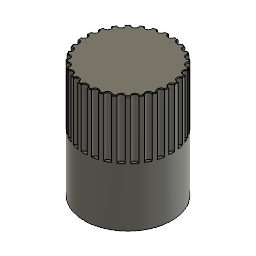
OpenMicroRotator (Autodesk Fusion 360 design; units mm, degrees)
Autodesk Fusion 360 part; units mm, degrees
sketch "Sketch1" plane through (0, 0, 0) normal (0, 1, 0) x (1, 0, 0)
  circle A0 centre (0, 0) radius 7.5
  dimension "d1" = 15
  constraint coincident A0.centre origin
  measures "d1" diameter of A0
extrude "Extrude1" add sketch "Sketch1" along normal blind 20
sketch "Sketch2" plane through (0, 0, 0) normal (0, -1, 0) x (1, 0, 0)
  circle A0 centre (0, 0) radius 7.5
  circle A1 centre (0, 0) radius 6.5
  dimension "d4" = 13
  constraint coincident A0.centre A1.centre
  measures "d4" diameter of A1
extrude "Extrude2" cut sketch "Sketch2" against normal blind 7 contours A1
sketch "Sketch3" plane through (0, 7, 0) normal (0, -1, 0) x (1, 0, 0)
  circle A0 centre (0, 0) radius 6.5
  circle A1 centre (0, 0) radius 3.025
  line L0 (-1.55, 2.5977) -> (-1.55, -2.5977)
  dimension "d7" = 6.05
  dimension "d8" = 1.55
  constraint coincident A0.centre A1.centre
  constraint coincident A1 L0.start
  constraint coincident A1 L0.end
  constraint vertical L0
  measures "d7" diameter of A1
  measures "d8" distance of A0.centre L0
extrude "Extrude3" cut sketch "Sketch3" against normal blind 10 contours A1 L0 picked at (0.0368, 0.8888)
sketch "Sketch4" plane through (0, 20, 0) normal (0, 1, 0) x (-1, 0, 0)
  circle A0 centre (0, 0) radius 7.5
  circle A1 centre (0, -7.5) radius 0.5
  circle A2 centre (1.6689, -7.312) radius 0.5
  circle A3 centre (3.2541, -6.7573) radius 0.5
  circle A4 centre (4.6762, -5.8637) radius 0.5
  circle A5 centre (5.8637, -4.6762) radius 0.5
  circle A6 centre (6.7573, -3.2541) radius 0.5
  circle A7 centre (7.312, -1.6689) radius 0.5
  circle A8 centre (7.5, 0) radius 0.5
  circle A9 centre (7.312, 1.6689) radius 0.5
  circle A10 centre (6.7573, 3.2541) radius 0.5
  circle A11 centre (5.8637, 4.6762) radius 0.5
  circle A12 centre (4.6762, 5.8637) radius 0.5
  circle A13 centre (3.2541, 6.7573) radius 0.5
  circle A14 centre (1.6689, 7.312) radius 0.5
  circle A15 centre (0, 7.5) radius 0.5
  circle A16 centre (-1.6689, 7.312) radius 0.5
  circle A17 centre (-3.2541, 6.7573) radius 0.5
  circle A18 centre (-4.6762, 5.8637) radius 0.5
  circle A19 centre (-5.8637, 4.6762) radius 0.5
  circle A20 centre (-6.7573, 3.2541) radius 0.5
  circle A21 centre (-7.312, 1.6689) radius 0.5
  circle A22 centre (-7.5, 0) radius 0.5
  circle A23 centre (-7.312, -1.6689) radius 0.5
  circle A24 centre (-6.7573, -3.2541) radius 0.5
  circle A25 centre (-5.8637, -4.6762) radius 0.5
  circle A26 centre (-4.6762, -5.8637) radius 0.5
  circle A27 centre (-3.2541, -6.7573) radius 0.5
  circle A28 centre (-1.6689, -7.312) radius 0.5
  dimension "d11" = 1
  dimension "d13" = 360
  constraint coincident A0 A1.centre
  measures "d11" diameter of A1
extrude "Extrude4" cut sketch "Sketch4" against normal blind 10 contours A0 A8 | A0 A9 | A0 A7 | A0 A10 | A0 A6 | A0 A11 | A0 A5 | A0 A12 | A0 A4 | A0 A13 | A0 A3 | A0 A14 | A0 A2 | A0 A15 | A0 A1 | A0 A16 | A0 A28 | A0 A17 | A0 A27 | A0 A18 | A0 A26 | A0 A19 | A0 A25 | A0 A20 | A0 A24 | A0 A21 | A0 A23 | A0 A22 picked at (7.3438, -0.1152) picked at (7.146, 1.6435) picked at (7.146, -1.6435) picked at (6.6117, 3.1705) picked at (6.6117, -3.1705) picked at (5.7404, 4.5622) picked at (5.7404, -4.5622) picked at (4.5622, 5.7404) picked at (4.5622, -5.7404) picked at (3.1705, 6.6117) picked at (3.1705, -6.6117) picked at (1.6198, 7.1514) picked at (1.6198, -7.1514) picked at (0.0122, 7.3325) picked at (0.0122, -7.3325) picked at (-1.6237, 7.1503) picked at (-1.6237, -7.1503) picked at (-3.1904, 6.6019) picked at (-3.1904, -6.6019) picked at (-4.5666, 5.7365) picked at (-4.5666, -5.7365) picked at (-5.7393, 4.5634) picked at (-5.7393, -4.5634) picked at (-6.6044, 3.1848) picked at (-6.6044, -3.1848) picked at (-7.1512, 1.6204) picked at (-7.1512, -1.6204) picked at (-7.3321, 0)
fillet "Fillet1" radius 0.1 56 edges at (-6.3504, 20, -3.9902) (-5.4728, 20, -4.3644) (-5.3033, 20, -5.3033) (-4.3644, 20, -5.4728) (-3.9902, 20, -6.3504) (-3.0372, 20, -6.3068) (-2.4771, 20, -7.0791) (-1.5576, 20, -6.8245) (-0.8397, 20, -7.4528) (0, 20, -7) (0.8397, 20, -7.4528) (1.5576, 20, -6.8245) (2.4771, 20, -7.0791) (3.0372, 20, -6.3068) (3.9902, 20, -6.3504) (4.3644, 20, -5.4728) (5.3033, 20, -5.3033) (5.4728, 20, -4.3644) (6.3504, 20, -3.9902) (6.3068, 20, -3.0372) (7.0791, 20, -2.4771) (6.8245, 20, -1.5576) (7.4528, 20, -0.8397) (7, 20, 0) (7.4528, 20, 0.8397) (6.8245, 20, 1.5576) (7.0791, 20, 2.4771) (6.3068, 20, 3.0372) (6.3504, 20, 3.9902) (5.4728, 20, 4.3644) (5.3033, 20, 5.3033) (4.3644, 20, 5.4728) (3.9902, 20, 6.3504) (3.0372, 20, 6.3068) (2.4771, 20, 7.0791) (1.5576, 20, 6.8245) (0.8397, 20, 7.4528) (0, 20, 7) (-0.8397, 20, 7.4528) (-1.5576, 20, 6.8245) (-2.4771, 20, 7.0791) (-3.0372, 20, 6.3068) (-3.9902, 20, 6.3504) (-4.3644, 20, 5.4728) (-5.3033, 20, 5.3033) (-5.4728, 20, 4.3644) (-6.3504, 20, 3.9902) (-6.3068, 20, 3.0372) (-7.0791, 20, 2.4771) (-6.8245, 20, 1.5576) (-7.4528, 20, 0.8397) (-7, 20, 0) (-7.4528, 20, -0.8397) (-6.8245, 20, -1.5576) (-7.0791, 20, -2.4771) (-6.3068, 20, -3.0372)
chamfer "Chamfer1" distance 1 angle 45 2 edges at (-1.55, 7, 0) (3.025, 7, 0)
fillet "Fillet2" radius 1 2 edges at (-1.55, 8, 0) (3.025, 8, 0)
